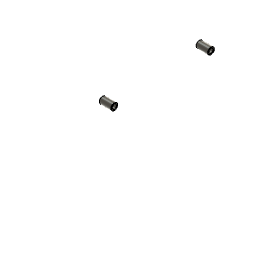
Spacers (Autodesk Fusion 360 design; units mm, degrees)
Autodesk Fusion 360 part; units mm, degrees
sketch "Sketch1" plane through (3, 0, 0) normal (1, 0, 0) x (0, 1, 0)
  circle A0 centre (15, 24.65) radius 1.4
  circle A1 centre (87, 27) radius 1.75
  circle A2 centre (3, 27) radius 1.75
  circle A3 centre (15, 2.85) radius 1.4
  circle A4 centre (15, 13.75) radius 2.5
  circle A5 centre (75, 13.75) radius 1.75
  line L0 (0, 30) -> (0, 0)
  line L1 (0, 0) -> (90, 0)
  line L2 (90, 0) -> (90, 30)
  line L3 (90, 30) -> (0, 30)
  circle A6 centre (3, 27) radius 1.75
  circle A7 centre (87, 27) radius 1.75
  circle A8 centre (3, 27) radius 1.75
  circle A9 centre (87, 27) radius 2.9
  circle A10 centre (3, 27) radius 2.9
  dimension "d20" = 3.5
  dimension "d21" = 5.8
  dimension "d123" = 5.8
  constraint concentric A2 A6
  constraint concentric A1 A7
  constraint concentric A6 A8
  constraint concentric A1 A9
  constraint concentric A6 A10
  measures "d20" diameter of A8
  measures "d21" diameter of A9
  measures "d123" diameter of A10
extrude "Extrude1" add sketch "Sketch1" along normal blind 10.4 contours A9 | A10 makes body 1 at (9.9333, 85.4266, 24.5639) makes body 2 at (9.9333, 5.8964, 26.8554)
chamfer "Chamfer1" distance 0.2 angle 45 4 edges at (13.4, 84.2963, 25.9513) (13.4, 85.3684, 27.6328) (3, 84.2963, 25.9513) (3, 85.3684, 27.6328) on bodies 1 2
chamfer "Chamfer1" distance 0.2 angle 45 3 edges at (3, 0.2963, 25.9513) (13.4, 1.3684, 27.6328) (13.4, 0.2963, 25.9513) on bodies 1 2
